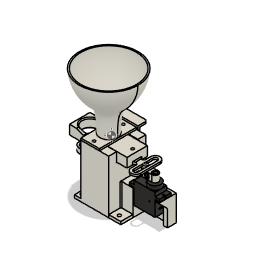
Skittle dispenser and sensor (Autodesk Fusion 360 design; units mm, degrees)
Autodesk Fusion 360 part; units mm, degrees
(part 1 of 2)
sketch "Sketch1" plane through (0, 0, 0) normal (0, 1, 0) x (1, 0, 0) in component "DoserSlider"
  line L0 (-31, 11) -> (31, 11)
  line L1 (31, 11) -> (31, -11)
  line L2 (31, -11) -> (-31, -11)
  line L3 (-31, -11) -> (-31, 11)
  circle A0 centre (-20, 0) radius 8.5
  line L4 (-31, -11) -> (31, 11) construction
  line L5 (0, 0) -> (-20, 0) construction
  circle A1 centre (26, 0) radius 1.5
  line L6 (0, 0) -> (26, 0) construction
  circle A2 centre (0, 0) radius 8.5 construction
  line L7 (37.5, 10.5) -> (37.5, -10.5)
  arc A3 (37.5, -10.5) -> (42.5, -10.5) centre (40, -10.5) ccw
  line L8 (42.5, -10.5) -> (42.5, 10.5)
  arc A4 (42.5, 10.5) -> (37.5, 10.5) centre (40, 10.5) ccw
  line L9 (40, 10.5) -> (40, -10.5) construction
  line L10 (40, 0) -> (31, 0) construction
  line L11 (35, 10.5) -> (35, -10.5)
  arc A5 (35, -10.5) -> (45, -10.5) centre (40, -10.5) ccw
  line L12 (45, -10.5) -> (45, 10.5)
  arc A6 (45, 10.5) -> (35, 10.5) centre (40, 10.5) ccw
  line L13 (40, 10.5) -> (40, -10.5) construction
  line L14 (31, 3) -> (35, 3)
  line L15 (31, -3) -> (35, -3)
  dimension "d13" = 17
  dimension "d15" = 22
  dimension "d16" = 20
  dimension "d17" = 5
  dimension "d18" = 3
  dimension "d19" = 17
  dimension "d20" = 20
  dimension "d21" = 11
  dimension "d202" = 5
  dimension "d203" = 9
  dimension "d204" = 21
  dimension "d205" = 10
  dimension "d206" = 6
  dimension "d207" = 3
  constraint horizontal L0
  constraint vertical L1
  constraint horizontal L2
  constraint vertical L3
  constraint midpoint L5.start L4
  constraint coincident L5.start L6.start
  constraint coincident A0.centre L5.end
  constraint horizontal L5
  constraint coincident A1.centre L6.end
  constraint parallel L5 L6
  constraint coincident L6 L5.start
  constraint tangent L7 A3
  constraint tangent A3 L8
  constraint parallel L7 L8
  constraint tangent L8 A4
  constraint tangent L7 A4
  constraint vertical L9
  constraint midpoint L9 L10.start
  constraint midpoint L1 L10.end
  constraint horizontal L10
  constraint tangent L11 A5
  constraint tangent A5 L12
  constraint parallel L11 L12
  constraint tangent L12 A6
  constraint tangent L11 A6
  constraint coincident A3.centre L9.end
  constraint parallel L9 L13
  constraint coincident A4.centre L9.start
  constraint coincident L1 L14.start
  constraint coincident L11 L14.end
  constraint perpendicular L11 L14
  constraint coincident L1 L15.start
  constraint coincident L11 L15.end
  constraint perpendicular L11 L15
  measures "d13" diameter of A0
  measures "d15" distance of L0.start L2.end
  measures "d16" distance of L5.start A0.centre
  measures "d17" distance of L1 A1.centre
  measures "d18" diameter of A1
  measures "d19" diameter of A2
  measures "d20" distance of A0.centre L5.start
  measures "d21" distance of L3 A0.centre
  measures "d202" distance of L7 L8
  measures "d203" distance of L10.start L10.end
  measures "d204" distance of A4.centre A3.centre
  measures "d205" distance of L11 L12
  measures "d206" distance of L14 L15
  measures "d207" distance of L10 L15
extrude "Extrude1" add sketch "Sketch1" along normal blind 10 contours L0 L1 L2 L3 makes body 1 in component "DoserSlider"
sketch "Sketch2" plane through (0, 0, 0) normal (0, -1, 0) x (1, 0, 0) in component "DoserSlider"
  circle A0 centre (-20, 0) radius 8.5
  circle A1 centre (26, 0) radius 1.5
  line L0 (31, 11) -> (-31, 11)
  line L1 (-31, 11) -> (-31, -11)
  line L2 (-31, -11) -> (31, -11)
  line L3 (31, -11) -> (31, 11)
  line L4 (-3, -2.5) -> (17, -2.5)
  arc A2 (17, -2.5) -> (17, 2.5) centre (17, 0) ccw
  line L5 (17, 2.5) -> (-3, 2.5)
  arc A3 (-3, 2.5) -> (-3, -2.5) centre (-3, 0) ccw
  line L6 (-3, 0) -> (17, 0) construction
  dimension "d65" = 20
  dimension "d66" = 5
  dimension "d67" = 3
  constraint tangent L4 A2
  constraint tangent A2 L5
  constraint parallel L4 L5
  constraint tangent L5 A3
  constraint tangent L4 A3
  constraint horizontal L6
  constraint coincident origin L6
  measures "d65" distance of A3.centre A2.centre
  measures "d66" distance of L4 L5
  measures "d67" distance of origin A3.centre
extrude "Extrude2" cut sketch "Sketch2" against normal blind 5 contours L4 A2 L5 A3 bodies 1 in component "DoserSlider"
chamfer "Chamfer1" distance 1 angle 45 2 edges at (-27.9248, 10, -3.0737) (-27.9248, 0, -3.0737) on bodies 1 in component "DoserSlider"
sketch "Sketch1 (2)" plane through (0, 0, 0) normal (0, 1, 0) x (1, 0, 0) in component "DoserBase"
  line L0 (-10, 20) -> (35, 20)
  line L1 (35, 20) -> (35, -20)
  line L2 (35, -20) -> (-10, -20)
  line L3 (-10, -20) -> (-10, 20)
  line L4 (-10, 11.5) -> (35, 11.5)
  line L5 (-10, -11.5) -> (35, -11.5)
  line L6 (0, -20) -> (0, 20) construction
  dimension "d28" = 40
  dimension "d29" = 8.5
  dimension "d30" = 8.5
  dimension "d54" = 10
  dimension "d55" = 35
  constraint horizontal L0
  constraint vertical L1
  constraint horizontal L2
  constraint vertical L3
  constraint coincident L3 L4.start
  constraint coincident L1 L4.end
  constraint perpendicular L1 L4
  constraint coincident L3 L5.start
  constraint coincident L1 L5.end
  constraint perpendicular L1 L5
  constraint coincident L2 L6.start
  constraint coincident L0 L6.end
  constraint perpendicular L0 L6
  constraint midpoint origin L6
  measures "d28" distance of L0.end L1.end
  measures "d29" distance of L2 L5
  measures "d30" distance of L0 L4
  measures "d54" distance of L3 L6
  measures "d55" distance of L1 L6
extrude "Extrude1'" add sketch "Sketch1 (2)" against normal blind 2 separate body makes body 2 in component "DoserBase"
extrude "Extrude2'" add sketch "Sketch1 (2)" along normal blind 10.5 contours L0 L1 L3 L4 | L1 L2 L3 L5 bodies 2 in component "DoserBase"
sketch "Sketch1 (3)" plane through (0, 10.5, 0) normal (0, 1, 0) x (-1, 0, 0) in component "Hopper"
  line L0 (10, -20) -> (10, -11.5)
  line L1 (10, -11.5) -> (-35, -11.5) construction
  line L2 (-35, -11.5) -> (-35, -20)
  line L3 (-35, -20) -> (10, -20)
  line L4 (10, 11.5) -> (10, 20)
  line L5 (10, 20) -> (-35, 20)
  line L6 (-35, 20) -> (-35, 11.5)
  line L7 (-35, 11.5) -> (10, 11.5) construction
  line L8 (-35, 11.5) -> (-35, -11.5)
  line L9 (10, -11.5) -> (10, 11.5)
  circle A0 centre (0, 0) radius 8
  line L10 (-10, -20) -> (-10, 20)
  dimension "d37" = 16
  dimension "d56" = 20
  constraint coincident L6.end L7.start
  constraint coincident L1.end L2.start
  constraint coincident L0.end L1.start
  constraint coincident L4.start L7.end
  constraint coincident A0.centre origin
  constraint coincident L3 L10.start
  constraint coincident L5 L10.end
  constraint perpendicular L5 L10
  measures "d37" diameter of A0
  measures "d56" distance of L9 L10
extrude "Extrude1''" add sketch "Sketch1 (3)" along normal blind 2 separate body contours L0 L3 L4 L5 L9 L10 makes body 3 in component "Hopper"
sketch "Sketch2 (2)" plane through (0, 0, 0) normal (0, 0, 1) x (1, 0, 0) in component "Hopper"
  line L0 (-8, 12.5) -> (8, 12.5)
  spline S0 degree 5 poles (8, 12.5) (8, 14.0765) (8.0277, 17.2259) (8.1523, 21.938) (8.5468, 28.0396) (9.735, 34.5699) (11.9017, 39.5191) (15.1786, 42.8048) (19.2244, 46.3465) (23.3886, 51.5557) (27.0347, 58.1658) (29.0417, 64.0264) (29.8258, 68.3446) (30, 71.1305) (30, 72.5) knots 0 0 0 0 0 0 0.1 0.2 0.3 0.4 0.5 0.6 0.7 0.8 0.9 1 1 1 1 1 1
  line L1 (8, 0) -> (8, 25)
  line L2 (0, 0) -> (0, 0.5)
  line L3 (0, 0.5) -> (0, 68.5) construction
  line L4 (9.6967, 37.1967) -> (20.3033, 47.8033)
  line L5 (30, 62.5) -> (30, 82.5)
  spline S1 degree 3 poles (9.5, 12.5) (9.5, 16.6886) (9.5998, 20.9098) (9.9239, 24.7925) (10.2195, 28.3342) (10.7207, 31.5443) (11.5284, 34.1184) (12.1469, 36.0897) (12.9314, 37.6615) (13.9182, 39.0059) (15.0071, 40.4897) (16.3987, 41.7681) (18.0186, 43.3428) (19.68, 44.9578) (21.5326, 46.9082) (23.2781, 49.2964) (25.928, 52.9218) (28.3407, 57.5142) (29.8342, 62.2902) (30.9024, 65.7061) (31.5, 69.18) (31.5, 72.5) knots 0 0 0 0 0.160486 0.160486 0.160486 0.306877 0.306877 0.306877 0.418988 0.418988 0.418988 0.542713 0.542713 0.542713 0.669601 0.669601 0.669601 0.862226 0.862226 0.862226 1 1 1 1
  line L6 (30, 72.5) -> (31.5, 72.5)
  line L7 (8, 12.5) -> (9.5, 12.5)
  point P0 (15, 42.5)
  dimension "d38" = 25
  dimension "d39" = 15
  dimension "d40" = 30
  dimension "d41" = 45
  dimension "d42" = 15
  dimension "d43" = 20
  dimension "d44" = 30
  dimension "d45" = 60
  dimension "d46" = 1.5
  constraint coincident L0.end S0.start
  constraint midpoint L0.end L1
  constraint vertical L1
  constraint coincident L2.start origin
  constraint perpendicular L0 L2
  constraint perpendicular L0 L3
  constraint midpoint P0 L4
  constraint midpoint S0.end L5
  constraint vertical L5
  constraint perpendicular L5 L6
  constraint perpendicular L1 L7
  measures "d38" distance of L1.start L1.end
  measures "d39" distance of P0 L3
  measures "d40" distance of L0 P0
  measures "d41" angle of L3 L4
  measures "d42" distance of L4.start L4.end
  measures "d43" distance of L5.start L5.end
  measures "d44" distance of S0.end L3
  measures "d45" distance of L0 S0.end
revolve "Revolve1" add sketch "Sketch2 (2)" angle 360 about axis through (0, 0.5, 0) along (0, 1, 0) contours S0 L5 S1 L7 | L5 S1 L6 bodies 3 in component "Hopper"
sketch "Sketch3" plane through (0, 12.5, 0) normal (0, 1, 0) x (-1, 0, 0) in component "Hopper"
  circle A0 centre (0, 0) radius 9.5
  line L0 (10, -20) -> (10, -11.5)
  line L1 (10, -11.5) -> (10, 11.5)
  line L2 (10, 11.5) -> (10, 20)
  line L3 (10, 20) -> (-10, 20)
  line L4 (-10, 20) -> (-10, -20)
  line L5 (-10, -20) -> (10, -20)
  line L6 (10, 15.75) -> (-10, 15.75) construction
  line L7 (10, -15.75) -> (-10, -15.75) construction
  circle A1 centre (0, 15.75) radius 1.5
  circle A2 centre (0, -15.75) radius 1.5
  circle A3 centre (0, 15.75) radius 0.75
  circle A4 centre (0, -15.75) radius 0.75
  dimension "d57" = 3
  dimension "d58" = 3
  dimension "d59" = 1.5
  dimension "d60" = 1.5
  constraint midpoint L2 L6.start
  constraint coincident L4 L6.end
  constraint perpendicular L4 L6
  constraint midpoint L0 L7.start
  constraint coincident L4 L7.end
  constraint perpendicular L4 L7
  constraint midpoint L6 A1.centre
  constraint midpoint L7 A2.centre
  constraint concentric A1 A3
  constraint concentric A2 A4
  measures "d57" diameter of A2
  measures "d58" diameter of A1
  measures "d59" diameter of A4
  measures "d60" diameter of A3
extrude "Extrude2''" cut sketch "Sketch3" against normal up to surface (2 mm away) contours A1 | A2 | A3 | A4 bodies 3 in component "Hopper"
extrude "Extrude3" cut sketch "Sketch3" against normal blind 10 contours A3 | A4 bodies 2 in component "DoserBase"
sketch "Sketch2 (3)" plane through (0, 0, 0) normal (0, 1, 0) x (-1, 0, 0) in component "DoserBase"
  line L0 (-35, -11.5) -> (10, -11.5)
  line L1 (10, -11.5) -> (10, 11.5)
  line L2 (10, 11.5) -> (-35, 11.5)
  line L3 (-35, 11.5) -> (-35, -11.5)
  arc A0 (-16.75, 2.5) -> (-16.75, -2.5) centre (-16.75, 0) ccw
  circle A1 centre (-16.75, 0) radius 2
  dimension "d70" = 4
  constraint concentric A0 A1
  measures "d70" diameter of A1
extrude "Extrude4" add sketch "Sketch2 (3)" along normal blind 3 contours A1 bodies 2 in component "DoserBase"
fillet "Fillet1" radius 1 1 edges at (18.6147, 3, -0.7232) on bodies 2 in component "DoserBase"
chamfer "Chamfer1'" distance 0.5 angle 45 1 edges at (18.6147, 0, 0.7232) on bodies 2 in component "DoserBase"
chamfer "Chamfer2" distance 0.5 angle 45 4 edges at (7, 0, -2.5) (-5.5, 0, 0) (7, 0, 2.5) (19.5, 0, 0) on bodies 1 in component "DoserSlider"
sketch "Sketch1 (4)" plane through (0, 0, 0) normal (0, 1, 0) x (1, 0, 0) in component "SensorPCB"
  line L0 (-10, 10) -> (10, 10)
  line L1 (10, 10) -> (10, -10)
  line L2 (10, -10) -> (-10, -10)
  line L3 (-10, -10) -> (-10, 10)
  line L4 (-10, -10) -> (10, 10) construction
  line L5 (0, -10) -> (0, 10) construction
  line L6 (-10, -7.5) -> (10, -7.5) construction
  circle A0 centre (-7.5, -7.5) radius 1.25
  circle A1 centre (7.5, -7.5) radius 1.25
  circle A2 centre (-7.62, 8.73) radius 0.75
  circle A3 centre (-5.08, 8.73) radius 0.75
  circle A4 centre (-2.54, 8.73) radius 0.75
  circle A5 centre (0, 8.73) radius 0.75
  circle A6 centre (2.54, 8.73) radius 0.75
  circle A7 centre (5.08, 8.73) radius 0.75
  circle A8 centre (7.62, 8.73) radius 0.75
  line L7 (-7.62, 8.73) -> (-10, 8.73)
  line L8 (7.62, 8.73) -> (10, 8.73)
  dimension "d77" = 20
  dimension "d78" = 20
  dimension "d79" = 15
  dimension "d80" = 2.5
  dimension "d81" = 2.5
  dimension "d82" = 2.5
  dimension "d83" = 1.5
  dimension "d86" = 2.54
  dimension "d87" = 0
  dimension "d88" = 1.27
  constraint horizontal L0
  constraint vertical L1
  constraint horizontal L2
  constraint vertical L3
  constraint midpoint origin L4
  constraint midpoint L2 L5.start
  constraint midpoint L0 L5.end
  constraint coincident L3 L6.start
  constraint coincident L1 L6.end
  constraint horizontal L6
  constraint coincident L6 A0.centre
  constraint symmetric L5 A0 A1
  constraint coincident A2.centre L7.start
  constraint coincident L3 L7.end
  constraint perpendicular L3 L7
  constraint coincident A8.centre L8.start
  constraint coincident L1 L8.end
  constraint perpendicular L1 L8
  constraint equal L7 L8
  measures "d77" distance of L0.start L2.end
  measures "d78" distance of L0.start L0.end
  measures "d79" distance of A0.centre A1.centre
  measures "d80" diameter of A0
  measures "d81" distance of L2 L6
  measures "d82" distance of L3 A0.centre
  measures "d83" diameter of A2
  measures "d88" distance of L0 L7
extrude "Extrude1'''" add sketch "Sketch1 (4)" along normal blind 1.2 separate body makes body 4 in component "SensorPCB"
fillet "Fillet1'" radius 1 4 edges at (10, 0.6, 10) (-10, 0.6, 10) (-10, 0.6, -10) (10, 0.6, -10) on bodies 4 in component "SensorPCB"
sketch "Sketch2 (4)" plane through (0, 1.2, 0) normal (0, 1, 0) x (-1, 0, 0) in component "SensorPCB"
  arc A0 (-10, -9) -> (-9, -10) centre (-9, -9) ccw
  line L0 (-9, -10) -> (9, -10)
  arc A1 (9, -10) -> (10, -9) centre (9, -9) ccw
  line L1 (10, -9) -> (10, 9)
  arc A2 (10, 9) -> (9, 10) centre (9, 9) ccw
  line L2 (9, 10) -> (-9, 10)
  arc A3 (-9, 10) -> (-10, 9) centre (-9, 9) ccw
  line L3 (-10, 9) -> (-10, -9)
  circle A4 centre (7.62, -8.73) radius 0.75
  circle A5 centre (-7.5, 7.5) radius 1.25
  circle A6 centre (2.54, -8.73) radius 0.75
  circle A7 centre (7.5, 7.5) radius 1.25
  circle A8 centre (-7.62, -8.73) radius 0.75
  circle A9 centre (0, -8.73) radius 0.75
  circle A10 centre (5.08, -8.73) radius 0.75
  circle A11 centre (-5.08, -8.73) radius 0.75
  circle A12 centre (-2.54, -8.73) radius 0.75
  line L4 (1, -1.25) -> (-1, -1.25)
  line L5 (-1, -1.25) -> (-1, 1.25)
  line L6 (-1, 1.25) -> (1, 1.25)
  line L7 (1, 1.25) -> (1, -1.25)
  line L8 (-1.5, -1.375) -> (-3.5, -1.375)
  line L9 (-3.5, -1.375) -> (-3.5, 1.375)
  line L10 (-3.5, 1.375) -> (-1.5, 1.375)
  line L11 (-1.5, 1.375) -> (-1.5, -1.375)
  line L12 (1, 1.25) -> (-1, -1.25) construction
  line L13 (-1.5, 1.375) -> (-3.5, -1.375) construction
  line L14 (-2.5, 0) -> (0, 0) construction
  line L15 (8.2885, -5.8633) -> (5.2885, -5.8633)
  line L16 (5.2885, -5.8633) -> (5.2885, -4.3633)
  line L17 (5.2885, -4.3633) -> (8.2885, -4.3633)
  line L18 (8.2885, -4.3633) -> (8.2885, -5.8633)
  line L19 (5.3165, 2.3816) -> (8.3165, 2.3816)
  line L20 (8.3165, 2.3816) -> (8.3165, 0.8816)
  line L21 (8.3165, 0.8816) -> (5.3165, 0.8816)
  line L22 (5.3165, 0.8816) -> (5.3165, 2.3816)
  line L23 (1.4928, -4.8493) -> (4.4928, -4.8493)
  line L24 (4.4928, -4.8493) -> (4.4928, -6.3493)
  line L25 (4.4928, -6.3493) -> (1.4928, -6.3493)
  line L26 (1.4928, -6.3493) -> (1.4928, -4.8493)
  line L27 (1.5924, -2.4927) -> (4.5924, -2.4927)
  line L28 (4.5924, -2.4927) -> (4.5924, -3.9927)
  line L29 (4.5924, -3.9927) -> (1.5924, -3.9927)
  line L30 (1.5924, -3.9927) -> (1.5924, -2.4927)
  line L31 (-4.4067, 4.374) -> (-1.4067, 4.374)
  line L32 (-1.4067, 4.374) -> (-1.4067, 2.874)
  line L33 (-1.4067, 2.874) -> (-4.4067, 2.874)
  line L34 (-4.4067, 2.874) -> (-4.4067, 4.374)
  line L35 (-0.4815, 4.2827) -> (2.5185, 4.2827)
  line L36 (2.5185, 4.2827) -> (2.5185, 2.7827)
  line L37 (2.5185, 2.7827) -> (-0.4815, 2.7827)
  line L38 (-0.4815, 2.7827) -> (-0.4815, 4.2827)
  line L39 (-4.8891, -0.7045) -> (-6.3891, -0.7045)
  line L40 (-6.3891, -0.7045) -> (-6.3891, 2.2955)
  line L41 (-6.3891, 2.2955) -> (-4.8891, 2.2955)
  line L42 (-4.8891, 2.2955) -> (-4.8891, -0.7045)
  line L43 (-7.0692, 2.3154) -> (-7.0692, -0.6846)
  line L44 (-7.0692, -0.6846) -> (-8.5692, -0.6846)
  line L45 (-8.5692, -0.6846) -> (-8.5692, 2.3154)
  line L46 (-8.5692, 2.3154) -> (-7.0692, 2.3154)
  line L47 (-6.3635, -2.5861) -> (-6.3635, -5.5861)
  line L48 (-6.3635, -5.5861) -> (-7.8635, -5.5861)
  line L49 (-7.8635, -5.5861) -> (-7.8635, -2.5861)
  line L50 (-7.8635, -2.5861) -> (-6.3635, -2.5861)
  line L51 (-2.7398, -5.6863) -> (-5.7398, -5.6863)
  line L52 (-5.7398, -5.6863) -> (-5.7398, -4.1863)
  line L53 (-5.7398, -4.1863) -> (-2.7398, -4.1863)
  line L54 (-2.7398, -4.1863) -> (-2.7398, -5.6863)
  line L55 (6.0638, -3.2947) -> (6.0638, -0.2947)
  line L56 (6.0638, -0.2947) -> (7.5638, -0.2947)
  line L57 (7.5638, -0.2947) -> (7.5638, -3.2947)
  line L58 (7.5638, -3.2947) -> (6.0638, -3.2947)
  line L59 (0.1718, -3.1838) -> (0.1718, -6.1838)
  line L60 (0.1718, -6.1838) -> (-1.3282, -6.1838)
  line L61 (-1.3282, -6.1838) -> (-1.3282, -3.1838)
  line L62 (-1.3282, -3.1838) -> (0.1718, -3.1838)
  dimension "d93" = 2
  dimension "d94" = 2.5
  dimension "d95" = 2.75
  dimension "d96" = 2
  dimension "d97" = 2.5
  dimension "d100" = 3
  dimension "d101" = 1.5
  constraint horizontal L4
  constraint vertical L5
  constraint horizontal L6
  constraint vertical L7
  constraint horizontal L8
  constraint vertical L9
  constraint horizontal L10
  constraint vertical L11
  constraint midpoint L14.end L12
  constraint midpoint L13 L14.start
  constraint coincident L14.end origin
  constraint horizontal L14
  constraint horizontal L15
  constraint vertical L16
  constraint horizontal L17
  constraint vertical L18
  constraint horizontal L21
  constraint vertical L22
  constraint horizontal L19
  constraint vertical L20
  constraint equal L16 L20
  constraint equal L15 L21
  constraint horizontal L25
  constraint vertical L26
  constraint horizontal L23
  constraint vertical L24
  constraint horizontal L29
  constraint vertical L30
  constraint horizontal L27
  constraint vertical L28
  constraint horizontal L33
  constraint vertical L34
  constraint horizontal L31
  constraint vertical L32
  constraint horizontal L37
  constraint vertical L38
  constraint horizontal L35
  constraint vertical L36
  constraint horizontal L39
  constraint vertical L40
  constraint horizontal L41
  constraint vertical L42
  constraint equal L16 L41
  constraint equal L15 L42
  constraint horizontal L44
  constraint vertical L45
  constraint horizontal L46
  constraint vertical L43
  constraint equal L16 L24
  constraint equal L16 L28
  constraint equal L15 L29
  constraint equal L15 L25
  constraint equal L15 L43
  constraint equal L16 L44
  constraint equal L25 L33
  constraint equal L18 L32
  constraint equal L16 L38
  constraint equal L15 L37
  constraint horizontal L48
  constraint vertical L49
  constraint horizontal L50
  constraint vertical L47
  constraint horizontal L51
  constraint vertical L52
  constraint horizontal L53
  constraint vertical L54
  constraint horizontal L58
  constraint vertical L55
  constraint horizontal L56
  constraint vertical L57
  constraint horizontal L60
  constraint vertical L61
  constraint horizontal L62
  constraint vertical L59
  measures "d93" distance of L5.end L6.end
  measures "d94" distance of L4.start L6.end
  measures "d95" distance of L8.end L9.end
  measures "d96" distance of L8.start L8.end
  measures "d97" distance of L14.start L14.end
  measures "d100" distance of L15.start L15.end
  measures "d101" distance of L15.start L17.end
extrude "Extrude2'''" add sketch "Sketch2 (4)" along normal blind 1 separate body contours L4 L5 L6 L7 | L8 L9 L10 L11 | L15 L16 L17 L18 | L19 L20 L21 L22 | L23 L24 L25 L26 | L27 L28 L29 L30 | L31 L32 L33 L34 | L35 L36 L37 L38 | L39 L40 L41 L42 | L43 L44 L45 L46 | L47 L48 L49 L50 | L51 L52 L53 L54 | L55 L56 L57 L58 | L59 L60 L61 L62 makes body 5 at (-0.3333, 1.2, -0.4167) makes body 6 at (2.1667, 1.2, -0.4583) makes body 7 at (-6.3165, 1.2, 1.8816) makes body 8 at (4.7398, 1.2, -5.1863) makes body 9 at (5.8891, 1.2, 1.2955) makes body 10 at (-2.4928, 1.2, -5.3493) makes body 11 at (-0.5185, 1.2, 3.7827) makes body 12 at (-7.2885, 1.2, -5.3633) makes body 13 at (7.3635, 1.2, -3.5861) makes body 14 at (7.5692, 1.2, 0.3154) makes body 15 at (-2.5924, 1.2, -2.9927) makes body 16 at (3.4067, 1.2, 3.874) makes body 17 at (-6.5638, 1.2, -1.2947) makes body 18 at (0.8282, 1.2, -4.1838) in component "SensorPCB"
sketch "Sketch1 (5)" plane through (0, 0, 0) normal (0, 1, 0) x (1, 0, 0) in component "SensorStand"
  line L0 (-20, 10) -> (20, 10)
  line L1 (20, 10) -> (20, -10)
  line L2 (20, -10) -> (-20, -10)
  line L3 (-20, -10) -> (-20, 10)
  line L4 (-15, 5) -> (15, 5) construction
  line L5 (15, 5) -> (15, -5) construction
  line L6 (15, -5) -> (-15, -5) construction
  line L7 (-15, -5) -> (-15, 5) construction
  line L8 (-20, -10) -> (20, 10) construction
  line L9 (15, -5) -> (-15, 5) construction
  circle A0 centre (-15, 5) radius 1.5
  circle A1 centre (-15, -5) radius 1.5
  circle A2 centre (15, -5) radius 1.5
  circle A3 centre (15, 5) radius 1.5
  dimension "d104" = 40
  dimension "d105" = 20
  dimension "d106" = 10
  dimension "d107" = 30
  dimension "d108" = 3
  dimension "d109" = 3
  dimension "d110" = 3
  dimension "d111" = 3
  constraint horizontal L0
  constraint vertical L1
  constraint horizontal L2
  constraint vertical L3
  constraint horizontal L4
  constraint vertical L5
  constraint horizontal L6
  constraint vertical L7
  constraint midpoint origin L8
  constraint midpoint origin L9
  constraint coincident L4.start L7.end
  constraint coincident L6.end L7.start
  constraint coincident L5.end L6.start
  constraint coincident L4.end L5.start
  measures "d104" distance of L0.start L0.end
  measures "d105" distance of L0.start L2.end
  measures "d106" distance of L4.start L6.end
  measures "d107" distance of L5.end L6.end
  measures "d108" diameter of A0
  measures "d109" diameter of A1
  measures "d110" diameter of A3
  measures "d111" diameter of A2
extrude "Extrude1''''" add sketch "Sketch1 (5)" along normal blind 3 separate body makes body 19 in component "SensorStand"
sketch "Sketch2 (5)" plane through (0, 3, 0) normal (0, 1, 0) x (-1, 0, 0) in component "SensorStand"
  circle A0 centre (15, -5) radius 1.5
  circle A1 centre (-15, -5) radius 1.5
  circle A2 centre (-15, 5) radius 1.5
  circle A3 centre (15, 5) radius 1.5
  line L0 (20, 10) -> (-20, 10)
  line L1 (-20, 10) -> (-20, -10)
  line L2 (-20, -10) -> (20, -10)
  line L3 (20, -10) -> (20, 10)
  line L4 (10, -10) -> (10, 10)
  line L5 (0, -10) -> (0, 10) construction
  line L6 (-10, -10) -> (-10, 10)
  line L7 (10, -4) -> (-10, -4)
  dimension "d114" = 20
  dimension "d120" = 6
  constraint coincident L2 L4.start
  constraint coincident L0 L4.end
  constraint perpendicular L0 L4
  constraint midpoint L2 L5.start
  constraint midpoint L0 L5.end
  constraint symmetric L4.start L5 L6.start
  constraint symmetric L4.end L5 L6.end
  constraint coincident L4 L7.start
  constraint coincident L6 L7.end
  constraint perpendicular L6 L7
  measures "d114" distance of L4 L6
  measures "d120" distance of L2 L7
extrude "Extrude2''''" add sketch "Sketch2 (5)" along normal blind 17 contours L0 L4 L6 L7 bodies 19 in component "SensorStand"
sketch "Sketch4" plane through (0, 20, 0) normal (0, 1, 0) x (-1, 0, 0) in component "SensorStand"
  line L0 (10, 10) -> (-10, 10)
  line L1 (-10, 10) -> (-10, -4)
  line L2 (-10, -4) -> (10, -4)
  line L3 (10, -4) -> (10, 10)
  circle A0 centre (7.5, 7.5) radius 1.25 construction
  circle A1 centre (-7.5, 7.5) radius 1.25 construction
  circle A2 centre (7.5, 7.5) radius 0.75
  circle A3 centre (-7.5, 7.5) radius 0.75
  line L4 (-10, -4) -> (-15, -4)
  line L5 (-15, -4) -> (-15, 10)
  line L6 (-15, 10) -> (-10, 10)
  line L7 (10, 10) -> (15, 10)
  line L8 (15, 10) -> (15, -4)
  line L9 (15, -4) -> (10, -4)
  line L10 (15, 0) -> (-15, 0) construction
  circle A4 centre (12.5, 0) radius 0.75
  line L11 (0, -4) -> (0, 10) construction
  circle A5 centre (-12.5, 0) radius 0.75
  dimension "d121" = 1.5
  dimension "d122" = 1.5
  dimension "d123" = 30
  dimension "d124" = 1.5
  dimension "d125" = 25
  dimension "d126" = 4
  constraint concentric A0 A2
  constraint concentric A1 A3
  constraint coincident L1.end L2.start
  constraint perpendicular L1 L4
  constraint perpendicular L4 L5
  constraint coincident L0.end L1.start
  constraint perpendicular L1 L6
  constraint coincident L0.start L3.end
  constraint perpendicular L3 L7
  constraint perpendicular L7 L8
  constraint coincident L2.end L3.start
  constraint horizontal L9
  constraint equal L4 L9
  constraint coincident L8 L10.start
  constraint coincident L5 L10.end
  constraint perpendicular L5 L10
  constraint coincident L10 A4.centre
  constraint midpoint L2 L11.start
  constraint midpoint L0 L11.end
  constraint symmetric A4 L11 A5
  measures "d121" diameter of A2
  measures "d122" diameter of A3
  measures "d123" distance of L5 L8
  measures "d124" diameter of A4
  measures "d125" distance of A4.centre A5.centre
  measures "d126" distance of L9 L10
extrude "Extrude4'" add sketch "Sketch4" against normal blind 2 contours L0 L1 L2 L3 | L3 L7 L8 L9 | L1 L4 L5 L6 | A2 | A3 | A4 | A5 bodies 19 in component "SensorStand"
chamfer "Chamfer1''" distance 10 distance2 5 2 edges at (10, 18, 3) (-10, 18, 3) measured on face at (10, 8, 0.6667) measured on face at (-10, 8, 0.6667) on bodies 19 in component "SensorStand"
extrude "Extrude5" cut sketch "Sketch4" against normal blind 4.5 contours A2 | A3 | A4 | A5 bodies 19 in component "SensorStand"
sketch "Sketch5" plane through (0, 20, 0) normal (0, 1, 0) x (-1, 0, 0) in component "SensorStand"
  circle A0 centre (7.5, 7.5) radius 0.75
  circle A1 centre (-7.5, 7.5) radius 0.75
  circle A2 centre (12.5, 0) radius 0.75
  circle A3 centre (-12.5, 0) radius 0.75
  line L0 (15, 10) -> (-15, 10)
  line L1 (-15, 10) -> (-15, -4)
  line L2 (-15, -4) -> (15, -4)
  line L3 (15, -4) -> (15, 10)
  line L4 (10.5, -4) -> (10.5, 10)
  line L5 (-10.5, -4) -> (-10.5, 10)
  dimension "d133" = 4.5
  dimension "d134" = 4.5
  constraint coincident L2 L4.start
  constraint coincident L0 L4.end
  constraint perpendicular L0 L4
  constraint coincident L2 L5.start
  constraint coincident L0 L5.end
  constraint perpendicular L0 L5
  measures "d133" distance of L1 L5
  measures "d134" distance of L3 L4
extrude "Extrude6" add sketch "Sketch5" along normal blind 3 contours L0 L2 L3 L4 | L0 L1 L2 L5 bodies 19 in component "SensorStand"
sketch "Sketch1 (6)" plane through (0, 23, 0) normal (0, 1, 0) x (-1, 0, 0) in component "SensorPlate"
  circle A0 centre (12.5, 0) radius 0.75 construction
  line L0 (15, -4) -> (15, 10)
  line L1 (15, 10) -> (10.5, 10)
  line L2 (10.5, 10) -> (10.5, -4) construction
  line L3 (10.5, -4) -> (15, -4) construction
  circle A1 centre (-12.5, 0) radius 0.75 construction
  line L4 (-10.5, -4) -> (-10.5, 10) construction
  line L5 (-10.5, 10) -> (-15, 10)
  line L6 (-15, 10) -> (-15, -4)
  line L7 (-15, -4) -> (-10.5, -4) construction
  line L8 (10.5, 10) -> (-10.5, 10)
  line L9 (-15, -4) -> (-15, -10)
  line L10 (-15, -10) -> (15, -10)
  line L11 (15, -10) -> (15, -4)
  circle A2 centre (12.5, 0) radius 1.5
  circle A3 centre (-12.5, 0) radius 1.5
  line L12 (4, -2) -> (-4, -2)
  line L13 (-4, -2) -> (-4, 2)
  line L14 (-4, 2) -> (4, 2)
  line L15 (4, 2) -> (4, -2)
  line L16 (4, 0) -> (-4, 0) construction
  line L17 (0, 0) -> (0, 2) construction
  dimension "d137" = 10
  dimension "d138" = 10
  dimension "d139" = 3
  dimension "d140" = 3
  dimension "d143" = 4
  dimension "d144" = 8
  dimension "d317" = 4
  constraint coincident L1.end L2.start
  constraint coincident L4.end L5.start
  constraint coincident L6.end L7.start
  constraint perpendicular L7 L9
  constraint perpendicular L9 L10
  constraint coincident L0.start L3.end
  constraint vertical L11
  constraint concentric A0 A2
  constraint concentric A1 A3
  constraint horizontal L12
  constraint vertical L13
  constraint horizontal L14
  constraint vertical L15
  constraint midpoint L15 L16.start
  constraint midpoint L13 L16.end
  constraint coincident L17.start L16
  constraint coincident L17.start origin
  constraint midpoint L14 L17.end
  constraint vertical L17
  measures "d137" distance of L17.start L8
  measures "d138" distance of L17.start L10
  measures "d139" diameter of A2
  measures "d140" diameter of A3
  measures "d143" distance of L12.start L14.end
  measures "d144" distance of L13.end L14.end
  measures "d317" distance of L17.start L13
extrude "Extrude1'''''" add sketch "Sketch1 (6)" along normal blind 1 separate body makes body 20 in component "SensorPlate"
fillet "Fillet1''" radius 1 4 edges at (-4, 23.5, -2) (4, 23.5, -2) (4, 23.5, 2) (-4, 23.5, 2) on bodies 20 in component "SensorPlate"
sketch "Sketch2 (6)" plane through (0, 24, 0) normal (0, 1, 0) x (-1, 0, 0) in component "SensorPlate"
  line L0 (-3, 2) -> (3, 2)
  arc A0 (4, 1) -> (3, 2) centre (3, 1) ccw
  line L1 (4, 1) -> (4, -1)
  arc A1 (3, -2) -> (4, -1) centre (3, -1) ccw
  line L2 (3, -2) -> (-3, -2)
  arc A2 (-4, -1) -> (-3, -2) centre (-3, -1) ccw
  line L3 (-4, -1) -> (-4, 1)
  arc A3 (-3, 2) -> (-4, 1) centre (-3, 1) ccw
  circle A4 centre (-12.5, 0) radius 1.5
  circle A5 centre (12.5, 0) radius 1.5
  line L4 (15, -10) -> (15, -4)
  line L5 (15, -4) -> (15, 10)
  line L6 (15, 10) -> (10.5, 10)
  line L7 (10.5, 10) -> (-10.5, 10)
  line L8 (-10.5, 10) -> (-15, 10)
  line L9 (-15, 10) -> (-15, -4)
  line L10 (-15, -4) -> (-15, -10)
  line L11 (-15, -10) -> (15, -10)
  circle A6 centre (0, 0) radius 8
  circle A7 centre (0, 0) radius 9
  line L12 (-9, 0) -> (-9, 10)
  line L13 (9, 0) -> (9, 10)
  line L14 (-8, 0) -> (-8, 10)
  line L15 (8, 10) -> (8, 0)
  line L16 (9, 8) -> (-9, 8)
  dimension "d148" = 16
  dimension "d149" = 1
  dimension "d314" = 2
  constraint coincident A6.centre A7.centre
  constraint coincident A7 L12.start
  constraint coincident L7 L12.end
  constraint perpendicular L7 L12
  constraint coincident A7 L13.start
  constraint coincident L7 L13.end
  constraint perpendicular L7 L13
  constraint tangent A7 L13
  constraint tangent A7 L12
  constraint coincident A6 L14.start
  constraint coincident L7 L14.end
  constraint perpendicular L7 L14
  constraint coincident L7 L15.start
  constraint coincident A6 L15.end
  constraint tangent A6 L15
  constraint perpendicular L7 L15
  constraint tangent A6 L14
  constraint coincident L13 L16.start
  constraint coincident L12 L16.end
  constraint perpendicular L12 L16
  measures "d148" diameter of A6
  measures "d149" distance of A6 A7
  measures "d314" distance of L7 L16
extrude "Extrude2'''''" add sketch "Sketch2 (6)" along normal blind 1 contours A7 L13 L15 L16 | A6 A7 L14 L15 | A7 L12 L14 L16 bodies 20 in component "SensorPlate"
sketch "Sketch1 (7)" plane through (0, 0, 0) normal (0, 0, 1) x (1, 0, 0) in component "Srevo_MG90S"
  line L0 (-11.375, -19.3) -> (11.375, -19.3)
  line L1 (11.375, -19.3) -> (11.375, -2.6)
  line L2 (11.375, -2.6) -> (16.25, -2.6)
  line L3 (16.25, -2.6) -> (16.25, 0)
  line L4 (16.25, 0) -> (11.375, 0)
  line L5 (11.375, 0) -> (11.375, 4.2)
  line L6 (11.375, 4.2) -> (-11.375, 4.2)
  line L7 (-11.375, 4.2) -> (-11.375, 0)
  line L8 (-11.375, 0) -> (-16.25, 0)
  line L9 (-16.25, 0) -> (-16.25, -2.6)
  line L10 (-16.25, -2.6) -> (-11.375, -2.6)
  line L11 (-11.375, -2.6) -> (-11.375, -19.3)
  line L12 (0, 4.2) -> (0, -19.3) construction
  line L13 (-11.375, 0) -> (-11.375, -2.6) construction
  line L14 (11.375, 0) -> (11.375, -2.6) construction
  line L15 (-11.375, 0) -> (11.375, 0) construction
  dimension "d1_1_1" = 22.75
  dimension "d2_1_1" = 23.5
  dimension "d3_1_1" = 32.5
  dimension "d4_1_1" = 4.2
  dimension "d5_1_1" = 2.6
  constraint horizontal L0
  constraint perpendicular L0 L1
  constraint perpendicular L1 L2
  constraint perpendicular L2 L3
  constraint perpendicular L3 L4
  constraint perpendicular L4 L5
  constraint perpendicular L5 L6
  constraint perpendicular L6 L7
  constraint perpendicular L7 L8
  constraint perpendicular L6 L9
  constraint perpendicular L9 L10
  constraint midpoint L6 L12.start
  constraint midpoint L0 L12.end
  constraint vertical L12
  constraint vertical L11
  constraint vertical L14
  constraint equal L4 L8
  constraint equal L3 L9
  constraint equal L5 L7
  constraint coincident origin L12
  constraint coincident origin L15
  measures "d1_1_1" distance of L0.start L0.end
  measures "d2_1_1" distance of L0 L6
  measures "d3_1_1" distance of L3 L9
  measures "d4_1_1" distance of L6.end L7.end
  measures "d5_1_1" distance of L8.end L9.end
extrude "Extrude1''''''" add sketch "Sketch1 (7)" along normal mid plane 12.5 separate body makes body 21 in component "Srevo_MG90S"
sketch "Sketch2 (7)" plane through (0, 0, 0) normal (0, 1, 0) x (-1, 0, 0) in component "Srevo_MG90S"
  line L0 (16.25, -6.25) -> (16.25, 6.25)
  line L1 (16.25, 6.25) -> (11.375, 6.25)
  line L2 (11.375, 6.25) -> (11.375, -6.25)
  line L3 (11.375, -6.25) -> (16.25, -6.25)
  line L4 (16.25, 0) -> (11.375, 0) construction
  line L5 (16.25, -0.6) -> (15.05, -0.6)
  line L6 (16.25, 0.6) -> (15.05, 0.6)
  arc A0 (15.05, 0.6) -> (15.05, -0.6) centre (14.25, 0) ccw
  dimension "d8_1_1" = 1.2
  dimension "d9_1_1" = 2
  dimension "d10_1_1" = 2
  constraint midpoint L0 L4.start
  constraint midpoint L2 L4.end
  constraint coincident L0 L5.start
  constraint perpendicular L0 L5
  constraint symmetric L4 L5.start L6.start
  constraint symmetric L4 L5.end L6.end
  constraint coincident A0.centre L4
  measures "d8_1_1" distance of L5 L6
  measures "d9_1_1" diameter of A0
  measures "d10_1_1" distance of L0 A0.centre
extrude "Extrude2''''''" cut sketch "Sketch2 (7)" against normal up to surface (2.6 mm away) contours L0 L5 L6 A0 bodies 21 in component "Srevo_MG90S"
mirror "Mirror1" about plane through (0, 0, 0) normal (1, 0, 0) of "Extrude2''''''" in component "Srevo_MG90S"
sketch "Sketch3 (2)" plane through (0, 4.2, 0) normal (0, 1, 0) x (-1, 0, 0) in component "Srevo_MG90S"
  line L0 (11.375, -6.25) -> (11.375, 6.25)
  line L1 (11.375, 6.25) -> (-11.375, 6.25)
  line L2 (-11.375, 6.25) -> (-11.375, -6.25)
  line L3 (-11.375, -6.25) -> (11.375, -6.25)
  circle A0 centre (5.125, 0) radius 6.25
  circle A1 centre (5.125, 0) radius 2.3
  circle A2 centre (-0.875, 0) radius 2.75
  line L4 (-0.875, -2.75) -> (-0.4875, -2.75)
  line L5 (-0.4875, 2.75) -> (-0.875, 2.75)
  line L6 (5.125, 0) -> (-0.875, 0) construction
  line L7 (-3.625, -6.25) -> (-3.625, 6.25) construction
  dimension "d15_1_1" = 4.6
  dimension "d16_1_1" = 5.5
  dimension "d1_1" = 15
  dimension "d2_1" = 6
  constraint tangent L3 A0
  constraint tangent L0 A0
  constraint tangent L1 A0
  constraint concentric A0 A1
  constraint coincident A2 L4.start
  constraint coincident A0 L4.end
  constraint horizontal L4
  constraint coincident A0 L5.start
  constraint coincident A2 L5.end
  constraint tangent A2 L5
  constraint tangent A2 L4
  constraint horizontal L5
  constraint coincident A0.centre A1.centre
  constraint coincident A2.centre L6.end
  constraint horizontal L6
  constraint coincident L3 L7.start
  constraint coincident L1 L7.end
  constraint perpendicular L1 L7
  constraint tangent A2 L7
  measures "d15_1_1" diameter of A1
  measures "d16_1_1" diameter of A2
  measures "d1_1" distance of L0 L7
  measures "d2_1" distance of A0.centre A2.centre
extrude "Extrude3'" add sketch "Sketch3 (2)" along normal blind 4.3 contours A0 A2 | A0 A2 L4 L5 | A0 A2 | A1 bodies 21 in component "Srevo_MG90S"
extrude "Extrude4''" add sketch "Sketch3 (2)" along normal blind 8 contours A1 bodies 21 in component "Srevo_MG90S"
fillet "Fillet1'''" radius 0.5 1 edges at (-2.9806, 12.2, -0.8317) on bodies 21 in component "Srevo_MG90S"
sketch "Sketch4 (2)" plane through (-11.375, 0, 0) normal (-1, 0, 0) x (0, 0, 1) in component "Srevo_MG90S"
  line L0 (-6.25, -19.3) -> (6.25, -19.3)
  line L1 (6.25, -19.3) -> (6.25, -2.6)
  line L2 (6.25, -2.6) -> (-6.25, -2.6)
  line L3 (-6.25, -2.6) -> (-6.25, -19.3)
  line L4 (-1.75, -12.8) -> (1.75, -12.8)
  line L5 (1.75, -12.8) -> (1.75, -14.05)
  line L6 (1.75, -14.05) -> (-1.75, -14.05)
  line L7 (-1.75, -14.05) -> (-1.75, -12.8)
  line L8 (0, -14.05) -> (0, -19.3) construction
  dimension "d24_1_1" = 1.25
  dimension "d25_1_1" = 3.5
  dimension "d26_1_1" = 5.25
  constraint horizontal L4
  constraint vertical L5
  constraint horizontal L6
  constraint vertical L7
  constraint midpoint L6 L8.start
  constraint midpoint L0 L8.end
  constraint vertical L8
  measures "d24_1_1" distance of L4.end L5.end
  measures "d25_1_1" distance of L4.start L4.end
  measures "d26_1_1" distance of L8.start L8.end
extrude "Extrude5'" cut sketch "Sketch4 (2)" against normal blind 1 contours L4 L5 L6 L7 bodies 21 in component "Srevo_MG90S"
sketch "Sketch5 (2)" plane through (0, 12.2, 0) normal (0, 1, 0) x (-1, 0, 0) in component "Srevo_MG90S"
  circle A0 centre (5.125, 0) radius 1.8
  circle A1 centre (5.125, 0) radius 1
  dimension "d29_1_1" = 2
  constraint concentric A0 A1
  measures "d29_1_1" diameter of A1
extrude "Extrude6'" cut sketch "Sketch5 (2)" against normal blind 2 contours A1 bodies 21 in component "Srevo_MG90S"
sketch "Sketch6" plane through (0, 0, 6.25) normal (0, 0, 1) x (1, 0, 0) in component "Srevo_MG90S"
  line L0 (-11.375, -2.6) -> (-11.375, -19.3)
  line L1 (-11.375, -19.3) -> (11.375, -19.3)
  line L2 (11.375, -19.3) -> (11.375, -2.6)
  line L3 (11.375, -2.6) -> (16.25, -2.6)
  line L4 (16.25, -2.6) -> (16.25, 0)
  line L5 (16.25, 0) -> (11.375, 0)
  line L6 (11.375, 0) -> (11.375, 4.2)
  line L7 (11.375, 4.2) -> (-5.125, 4.2)
  line L8 (-5.125, 4.2) -> (-11.375, 4.2)
  line L9 (-11.375, 4.2) -> (-11.375, 0)
  line L10 (-11.375, 0) -> (-16.25, 0)
  line L11 (-16.25, 0) -> (-16.25, -2.6)
  line L12 (-16.25, -2.6) -> (-11.375, -2.6)
  line L13 (-6.125, 12.2) -> (-4.125, 12.2)
  line L14 (-5.125, 12.2) -> (-5.125, -19.3) construction
  line L15 (0.4875, 8.5) -> (-11.375, 8.5)
  line L16 (-11.375, 8.5) -> (-11.375, -19.3) construction
  line L17 (-11.375, -7.4) -> (11.375, -7.4) construction
  circle A0 centre (-5.125, -7.4) radius 0.5
  line L18 (-11.375, -5.4) -> (11.375, -5.4) construction
  dimension "d80_1" = 31.5
  dimension "d82_1" = 3.7
  dimension "d83_1" = 1
  dimension "d240_1" = 2
  constraint midpoint L13 L14.start
  constraint coincident L1 L14.end
  constraint perpendicular L1 L14
  constraint coincident L1 L0.end
  constraint perpendicular L1 L16
  constraint coincident L2 L17.end
  constraint perpendicular L2 L17
  constraint coincident L15.end L16.start
  constraint coincident L14 A0.centre
  constraint coincident L17 A0.centre
  constraint midpoint L16 L18.start
  constraint coincident L2 L18.end
  constraint perpendicular L2 L18
  measures "d80_1" distance of L14.start L14.end
  measures "d82_1" distance of L13 L15
  measures "d83_1" diameter of A0
  measures "d240_1" distance of L17 L18
extrude "Extrude7" cut sketch "Sketch6" against normal blind 0.5 contours A0 bodies 21 in component "Srevo_MG90S"
mirror "Mirror2" about plane through (0, 0, 0) normal (0, 0, 1) of "Extrude7" in component "Srevo_MG90S"
sketch "Sketch1 (8)" plane through (0, 0, 0) normal (0, 1, 0) x (1, 0, 0) in component "SliderSwing"
  circle A0 centre (0, 0) radius 2.35
  circle A1 centre (0, 0) radius 10 construction
  circle A2 centre (-10, 0) radius 2.25
  line L0 (-10, -3.5) -> (0, -3.5)
  arc A3 (0, -3.5) -> (0, 3.5) centre (0, 0) ccw
  line L1 (0, 3.5) -> (-10, 3.5)
  arc A4 (-10, 3.5) -> (-10, -3.5) centre (-10, 0) ccw
  line L2 (-10, 0) -> (0, 0) construction
  circle A5 centre (0, 0) radius 1.4
  circle A6 centre (0, 0) radius 3.5
  dimension "d161" = 4.7
  dimension "d162" = 20
  dimension "d164" = 4.5
  dimension "d165" = 7
  dimension "d166" = 2.8
  constraint concentric A0 A1
  constraint coincident A1 A2.centre
  constraint tangent L0 A3
  constraint tangent A3 L1
  constraint parallel L0 L1
  constraint tangent L1 A4
  constraint tangent L0 A4
  constraint coincident A0.centre A1.centre
  constraint coincident A2.centre A4.centre
  constraint horizontal L2
  constraint concentric A3 A5
  constraint concentric A0 A6
  constraint coincident A3.end A6
  measures "d161" diameter of A0
  measures "d162" diameter of A1
  measures "d164" diameter of A2
  measures "d165" distance of L0 L1
  measures "d166" diameter of A5
extrude "Extrude1'''''''" add sketch "Sketch1 (8)" along normal blind 5 separate body contours A0 | A2 | L0 L1 A4 A6 | A3 A6 makes body 22 in component "SliderSwing"
extrude "Extrude4'''" cut sketch "Sketch1 (8)" along normal blind 3 contours A0 bodies 22 in component "SliderSwing"
chamfer "Chamfer3" distance 0.95 angle 45 1 edges at (-1.3053, 3, -0.5063) on bodies 22 in component "SliderSwing"
sketch "Sketch2 (8)" plane through (0, 5, 0) normal (0, 1, 0) x (-1, 0, 0) in component "SliderSwing"
  circle A0 centre (0, 0) radius 1.4
  arc A1 (0, 3.5) -> (0, -3.5) centre (0, 0) ccw
  line L0 (0, -3.5) -> (10, -3.5)
  arc A2 (10, -3.5) -> (10, 3.5) centre (10, 0) ccw
  line L1 (10, 3.5) -> (0, 3.5)
  circle A3 centre (0, 0) radius 2.5
  dimension "d181" = 5
  constraint concentric A0 A3
  measures "d181" diameter of A3
extrude "Extrude5''" add sketch "Sketch2 (8)" along normal blind 2 contours A1 L0 A2 L1 bodies 22 in component "SliderSwing"
sketch "Sketch3 (3)" plane through (0, 7, 0) normal (0, 1, 0) x (-1, 0, 0) in component "SliderSwing"
  circle A0 centre (0, 0) radius 2.5
  line L0 (10, 3.5) -> (0, 3.5)
  arc A1 (0, 3.5) -> (0, -3.5) centre (0, 0) ccw
  line L1 (0, -3.5) -> (10, -3.5)
  arc A2 (10, -3.5) -> (10, 3.5) centre (10, 0) ccw
  circle A3 centre (10, 0) radius 2.25
  dimension "d184" = 4.5
  constraint concentric A2 A3
  measures "d184" diameter of A3
extrude "Extrude6''" add sketch "Sketch3 (3)" along normal blind 4 contours A3 bodies 22 in component "SliderSwing"
fillet "Fillet1''''" radius 1 1 edges at (-7.9023, 11, -0.8136) on bodies 22 in component "SliderSwing"
chamfer "Chamfer5" distance 0.5 distance2 0.5 1 edges at (2.3308, 7, 0.904) measured on face at (-3.8529, 7, 2.9849) on bodies 22 in component "SliderSwing"
chamfer "Chamfer6" distance 0.2 distance2 2 1 edges at (-2.191, 0, 0.8498) measured on face at (-7.45, 0, 0) on bodies 22 in component "SliderSwing"
sketch "Sketch4 (3)" plane through (0, 0, 3.5) normal (0, 0, 1) x (1, 0, 0) in component "SliderSwing"
  line L0 (-10, 0) -> (0, 0)
  line L1 (0, 0) -> (0, 7)
  line L2 (0, 7) -> (-10, 7)
  line L3 (-10, 7) -> (-10, 0)
  line L4 (-7.9338, 3.5871) -> (-3.7137, 3.5871) construction
  line L5 (-3.7137, 3.5871) -> (-3.7137, 7.4274) construction
  line L6 (-3.7137, 7.4274) -> (-7.9338, 7.4274) construction
  line L7 (-7.9338, 7.4274) -> (-7.9338, 3.5871) construction
  dimension "d193" = 5
  text T0 "G" font "Arial" height 5 bold align left top in box 4.2201 x 3.8403 at (-7.9338, 3.5871) x (1, 0) y (0, 1) spacing 1 kerned
extrude "Extrude7'" add sketch "Sketch4 (3)" along normal blind 0.2 text T0 bodies 22 in component "SliderSwing"
chamfer "Chamfer1'''" distance 2 distance2 1 3 edges at (-9, 24, 4) (0, 24, -9) (9, 24, 4) measured on face at (-1, 24, 6) measured on face at (-1, 24, 6) measured on face at (-1, 24, 6) on bodies 20 in component "SensorPlate"
extrude "Extrude3''" add sketch "Sketch1" along normal blind 2 contours L1 L11 L14 L15 | L11 A5 L12 A6 bodies 1 in component "DoserSlider"
fillet "Fillet2" radius 2 4 edges at (31, 1, -3) (31, 1, 3) (35, 1, 3) (35, 1, -3) on bodies 1 in component "DoserSlider"
chamfer "Chamfer3'" distance 1 angle 45 1 edges at (31, 2, 0) on bodies 1 in component "DoserSlider"
sketch "Sketch3 (4)" plane through (0, 0, 11) normal (0, 0, 1) x (1, 0, 0) in component "DoserSlider"
  line L0 (-31, 0) -> (31, 0)
  line L1 (31, 0) -> (31, 10)
  line L2 (31, 10) -> (-31, 10)
  line L3 (-31, 10) -> (-31, 0)
  line L4 (-8.5, 10) -> (-16, 7)
  line L5 (-16, 7) -> (-23.5, 10)
  line L6 (-28.5, 9) -> (-11.5, 9) construction
  line L7 (-11.5, 1) -> (-28.5, 1) construction
  line L8 (-11.5, 9) -> (-11.5, 1) construction
  line L9 (-28.5, 9) -> (-28.5, 1) construction
  dimension "d213" = 3
  dimension "d214" = 15
  dimension "d215" = 3
  constraint coincident L2 L4.start
  constraint coincident L2 L5.end
  constraint coincident L6.end L8.start
  constraint coincident L7.start L8.end
  constraint coincident L6.start L9.start
  constraint coincident L7.end L9.end
  constraint equal L4 L5
  measures "d213" distance of L4.start L8
  measures "d214" distance of L4.start L5.end
  measures "d215" distance of L2 L4.end
extrude "Extrude4''''" cut sketch "Sketch3 (4)" against normal up to surface (22 mm away) contours L2 L4 L5 bodies 1 in component "DoserSlider"
extrude "Extrude5'''" cut 1 faces at (35, 2.8333, -17.1667) along direction (-1, 0, 0) blind 15 on bodies 2 bodies 2 in component "DoserBase"
extrude "Extrude6'''" add 1 faces at (0, -2, -6.6667) along direction (0, -1, 0) blind 45 on bodies 2 bodies 2 in component "DoserBase"
sketch "Sketch3 (5)" plane through (20, 0, 0) normal (1, 0, 0) x (0, 0, -1) in component "DoserBase"
  line L0 (11.5, 0) -> (-11.5, 0)
  line L1 (-11.5, 0) -> (-11.5, 10.5)
  line L2 (-11.5, 10.5) -> (-20, 10.5)
  line L3 (-20, 10.5) -> (-20, -47)
  line L4 (-20, -47) -> (20, -47)
  line L5 (20, -47) -> (20, 10.5)
  line L6 (20, 10.5) -> (11.5, 10.5)
  line L7 (11.5, 10.5) -> (11.5, 0)
  line L8 (6.25, -18.8) -> (-6.25, -18.8)
  line L9 (-20, -19.3) -> (20, -19.3)
  dimension "d226" = 0.5
  constraint coincident L3 L9.start
  constraint coincident L5 L9.end
  constraint perpendicular L5 L9
  measures "d226" distance of L8 L9
extrude "Extrude7''" add sketch "Sketch3 (5)" along normal up to surface (41.125 mm away) contours L3 L4 L5 L9 bodies 2 in component "DoserBase"
sketch "Sketch4 (4)" plane through (0, -19.3, 0) normal (0, 1, 0) x (-1, 0, 0) in component "DoserBase"
  line L0 (-61.125, 20) -> (-61.125, -20)
  line L1 (-61.125, -20) -> (-20, -20)
  line L2 (-20, -20) -> (-20, 20)
  line L3 (-20, 20) -> (-61.125, 20)
  line L4 (-33.5, 6.25) -> (-33.5, -6.25) construction
  line L5 (-33.5, -6.25) -> (-56.25, -6.25) construction
  line L6 (-56.25, -6.25) -> (-56.25, 6.25) construction
  line L7 (-56.25, 6.25) -> (-33.5, 6.25) construction
  line L8 (-56.75, 6.75) -> (-33, 6.75)
  line L9 (-33, 6.75) -> (-33, -6.75)
  line L10 (-33, -6.75) -> (-56.75, -6.75)
  line L11 (-56.75, -6.75) -> (-56.75, 6.75)
  arc A0 (-59.925, -0.6) -> (-59.925, 0.6) centre (-59.125, 0) ccw construction
  arc A1 (-29.825, 0.6) -> (-29.825, -0.6) centre (-30.625, 0) ccw construction
  circle A2 centre (-30.625, 0) radius 0.75
  circle A3 centre (-59.125, 0) radius 0.75
  line L12 (-56.75, 6.75) -> (-61.125, 6.75)
  line L13 (-33, 6.75) -> (-20, 6.75)
  line L14 (-61.125, -11.75) -> (-20, -11.75)
  dimension "d229" = -0.5
  dimension "d230" = 1.5
  dimension "d231" = 1.5
  dimension "d241" = 5
  constraint concentric A1 A2
  constraint concentric A0 A3
  constraint coincident L0 L12.end
  constraint perpendicular L0 L12
  constraint coincident L2 L13.end
  constraint perpendicular L2 L13
  constraint coincident L0 L14.start
  constraint coincident L2 L14.end
  constraint perpendicular L2 L14
  measures "d230" diameter of A2
  measures "d231" diameter of A3
  measures "d241" distance of L10 L14
extrude "Extrude8" cut sketch "Sketch4 (4)" against normal up to surface (27.7 mm away) contours L0 L2 L3 L8 L12 L13 | L0 L1 L2 L14 | L8 L9 L10 L11 bodies 2 in component "DoserBase"
sketch "Sketch5 (3)" plane through (61.125, 0, 0) normal (1, 0, 0) x (0, 0, -1) in component "DoserBase"
  line L0 (-6.75, -19.3) -> (-6.75, -47)
  line L1 (-6.75, -47) -> (11.75, -47)
  line L2 (11.75, -19.3) -> (-6.75, -19.3)
  line L3 (-1.75, -29) -> (1.75, -29) construction
  line L4 (-6.75, -20) -> (2.25, -20)
  line L5 (2.25, -20) -> (2.25, -47)
  line L6 (-6.75, -20) -> (2.25, -29)
  line L7 (1.75, -29) -> (2.25, -29) construction
  line L8 (11.75, -47) -> (11.75, -19.3)
  dimension "d234" = 9
  dimension "d236" = 45
  constraint coincident L0 L4.start
  constraint perpendicular L0 L4
  constraint coincident L1 L5.end
  constraint perpendicular L1 L5
  constraint coincident L5 L6.end
  constraint coincident L3.end L7.start
  constraint horizontal L7
  measures "d234" distance of L0 L5
  measures "d236" angle of L4 L6
extrude "Extrude9" cut sketch "Sketch5 (3)" against normal up to surface (4.375 mm away) contours L0 L1 L5 L6 bodies 2 in component "DoserBase"
extrude "Extrude10" cut sketch "Sketch4 (4)" against normal blind 6 contours A2 | A3 bodies 2 in component "DoserBase"